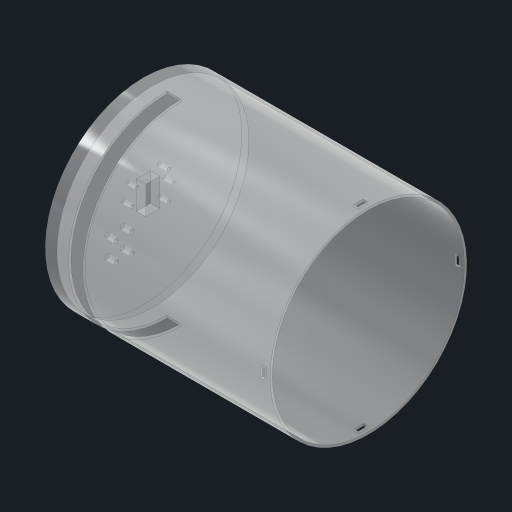
# Autodesk Inventor part: OUTK_001_ChipBucket
Saved by Autodesk Inventor 2024.2 (Build 282272000, 272)
## iProperties
Created: 2024-11-24
Part Number: OUTK_001_ChipBucket
Material: Polycarbonate, Clear
Document SubType Name: Modeling
Designer: Bryan
Density: 1.2 g/cm^3
Appearance: Polycarbonate - Clear
Mass: 1651.38 g
Surface Area: 5531.68 cm^2
Volume: 1376.15 cm^3
Author: Bryan
Autodesk Inventor part; units mm, degrees
ref_plane "YZ Plane" through (0, 0, 0) normal (1, 0, 0) x (0, 1, 0)
ref_plane "XZ Plane" through (0, 0, 0) normal (0, 1, 0) x (-1, 0, 0)
ref_plane "XY Plane" through (0, 0, 0) normal (0, 0, 1) x (1, 0, 0)
sketch "Sketch1" plane through (0, 0, 0) normal (1, 0, 0) x (0, 1, 0)
  circle A0 centre (0, 0) radius 133.35
  dimension "d0" = 266.7
  constraints: 1 centre point, 1 coincident
  measures "d0" diameter of A0
extrude "Extrusion1" add sketch "Sketch1" along normal mid plane 304.8
sketch "Sketch2" plane through (152.4, 0, 0) normal (1, 0, 0) x (0, 0, -1)
  circle A0 centre (0, 0) radius 130.175
  dimension "d3" = 260.35
  constraints: 1 centre point, 1 coincident
  measures "d3" diameter of A0
extrude "Extrusion2" cut sketch "Sketch2" against normal blind 292.1
sketch "Sketch3" plane through (0, 0, 0) normal (0, 0, 1) x (1, 0, 0)
  line L0 (-139.7, 130.175) -> (-139.7, -130.175) projected
  line L1 (152.4, 130.175) -> (152.4, -130.175) projected
  line L2 (152.4, 130.175) -> (-139.7, 130.175) projected
  line L3 (152.4, -130.175) -> (-139.7, -130.175) projected
  line L4 (-120.65, 130.175) -> (-120.65, -130.175)
  line L5 (-101.6, -130.175) -> (-101.6, 130.175)
  point P0 (0, 0)
  dimension "d6" = 19.05
  dimension "d7" = 19.05
  constraints: 4 end point, 4 point on line, 1 parallel, 1 vertical
  measures "d6" distance between parallel lines of L0 L4
  measures "d7" distance between parallel lines of L4 L5
extrude "Extrusion3" cut sketch "Sketch3" along normal blind 266.7 contours L2 L5 L3 L4
sketch "Sketch4" plane through (0, 0, 0) normal (0, 1, 0) x (-1, 0, 0)
  line L0 (120.65, 0) -> (101.6, 0) projected
  line L1 (120.65, 0) -> (120.65, 28.9256) projected
  line L2 (101.6, 0) -> (101.6, 28.9256) projected
  line L3 (101.6, 28.9256) -> (120.65, 28.9256) projected
  point P0 (0, 0)
extrude "Extrusion4" cut sketch "Sketch4" along normal through all both and the other way through all
sketch "Sketch5" plane through (0, 0, 0) normal (0, 1, 0) x (-1, 0, 0)
  line L0 (-139.065, 6.35) -> (-144.78, 6.35)
  line L1 (-144.78, 6.35) -> (-144.78, -6.35)
  line L2 (-144.78, -6.35) -> (-139.065, -6.35)
  line L3 (-139.065, -6.35) -> (-139.065, 6.35)
  line L4 (-152.4, 133.35) -> (-152.4, -133.35) projected
  point P0 (0, 0)
  point P1 (-139.065, 0)
  dimension "d12" = 5.715
  dimension "d13" = 12.7
  dimension "d14" = 7.62
  constraints: 8 end point, 2 parallel, 1 horizontal, 1 horizontal alignment, 1 midpoint, 1 perpendicular
  measures "d12" distance of L2.end L1.end
  measures "d13" distance of L1.end L0.end
  measures "d14" distance between parallel lines of L4 L1
extrude "Extrusion5" cut sketch "Sketch5" along normal through all both and the other way through all
sketch "Sketch6" plane through (0, 0, 0) normal (0, 0, 1) x (1, 0, 0)
  line L0 (139.065, 6.35) -> (144.78, 6.35)
  line L1 (144.78, 6.35) -> (144.78, -6.35)
  line L2 (144.78, -6.35) -> (139.065, -6.35)
  line L3 (139.065, -6.35) -> (139.065, 6.35)
  line L4 (152.4, -133.35) -> (152.4, 133.35) projected
  point P0 (0, 0)
  point P1 (139.065, 0)
  dimension "d17" = 5.715
  dimension "d18" = 12.7
  dimension "d19" = 7.62
  constraints: 8 end point, 2 parallel, 1 horizontal, 1 horizontal alignment, 1 midpoint, 1 perpendicular
  measures "d17" distance of L1.end L2.end
  measures "d18" distance of L0.end L1.end
  measures "d19" distance between parallel lines of L4 L1
extrude "Extrusion6" cut sketch "Sketch6" along normal through all both and the other way through all
sketch "Sketch8" plane through (-152.4, 0, 0) normal (-1, 0, 0) x (0, 0, 1)
  line L0 (-9.525, -19.05) -> (9.525, -19.05)
  line L1 (9.525, -19.05) -> (9.525, 19.05)
  line L2 (9.525, 19.05) -> (-9.525, 19.05)
  line L3 (-9.525, 19.05) -> (-9.525, -19.05)
  circle A0 centre (28.575, -27.1526) radius 3.2512
  circle A1 centre (28.575, -52.5526) radius 3.2512
  circle A2 centre (49.4284, -27.1526) radius 3.2512
  circle A3 centre (49.4284, -52.5526) radius 3.2512
  line L4 (-9.525, -14.4526) -> (9.525, -14.4526) construction
  line L5 (0, -14.4526) -> (0, -65.2526) construction
  line L6 (28.575, -27.1526) -> (28.575, -52.5526) construction
  line L7 (-6.35, -15.875) -> (-6.35, 15.875) construction
  line L8 (-6.35, 15.875) -> (6.35, 15.875) construction
  line L9 (6.35, 15.875) -> (6.35, -15.875) construction
  line L10 (6.35, -15.875) -> (-6.35, -15.875) construction
  line L11 (-6.35, -8.1026) -> (-2.3812, -4.1338) construction
  line L12 (-2.3812, -4.1338) -> (-2.3812, 8.5662) construction
  line L13 (6.35, 12.5349) -> (2.3813, 8.5662) construction
  line L14 (2.3813, 8.5662) -> (2.3813, -4.1338) construction
  line L15 (2.3813, -4.1338) -> (6.35, -8.1026) construction
  line L16 (0, -15.875) -> (0, 15.875) construction
  line L17 (-2.3812, 8.5662) -> (-6.35, 12.5349) construction
  line L18 (2.3813, 8.5662) -> (21.4312, 8.5662) construction
  line L19 (21.4312, 8.5662) -> (21.4312, -4.1339) construction
  line L20 (21.4312, -4.1339) -> (2.3813, -4.1338) construction
  line L21 (2.3813, -4.1338) -> (2.3813, 8.5662) construction
  line L22 (-2.3812, 8.5662) -> (-21.4312, 8.5661) construction
  line L23 (-21.4312, 8.5661) -> (-21.4312, -4.1338) construction
  line L24 (-21.4312, -4.1338) -> (-2.3812, -4.1338) construction
  line L25 (-2.3812, -4.1338) -> (-2.3812, 8.5662) construction
  line L26 (-15.0812, 14.9162) -> (-8.7312, 14.9162) construction
  line L27 (-8.7312, 14.9162) -> (-8.7312, -10.4839) construction
  line L28 (-8.7312, -10.4839) -> (-15.0812, -10.4839) construction
  line L29 (-15.0812, -10.4839) -> (-15.0812, 14.9162) construction
  line L30 (-21.4312, 2.2161) -> (-15.0812, 2.2161) construction
  circle A4 centre (-21.4312, -16.8338) radius 2.4892
  circle A5 centre (-27.7812, 2.2161) radius 2.4892
  circle A6 centre (-21.4312, 21.2662) radius 2.4892
  circle A7 centre (21.4312, -16.8338) radius 2.4892
  circle A8 centre (27.7812, 2.2161) radius 2.4892
  circle A9 centre (21.4312, 21.2662) radius 2.4892
  point P0 (0, 0)
  point P1 (28.575, -39.8526)
  point P2 (0, -39.8526)
  point P3 (-2.3813, 2.2162)
  point P4 (0, 0)
  point P5 (0, 19.05)
  point P6 (-9.525, 0)
  point P7 (-11.9062, 14.9162)
  point P8 (-11.9062, 8.5662)
  point P9 (-11.9062, -10.4839)
  point P10 (-18.2562, 2.2161)
  dimension "d22" = 19.05
  dimension "d23" = 38.1
  dimension "d24" = 6.5024
  dimension "d25" = 25.4
  dimension "d26" = 20.8534
  dimension "d28" = 19.05
  dimension "d31" = 4.5974
  dimension "d32" = 50.8
  dimension "d35" = 3.175
  dimension "d36" = 3.175
  dimension "d37" = 3.175
  dimension "d38" = 3.175
  dimension "d39" = 3.9688
  dimension "d40" = 12.7
  dimension "d41" = 45
  dimension "d42" = 45
  dimension "d44" = 19.05
  dimension "d45" = 6.35
  dimension "d46" = 25.4
  dimension "d47" = 7.7724
  dimension "d56" = 12.7
  dimension "d57" = 4.9784
  dimension "d58" = 6.35
  dimension "d59" = 19.05
  dimension "d60" = 6.35
  constraints: 62 end point, 15 midpoint, 10 centre point, 8 horizontal, 8 horizontal alignment, 8 parallel, 6 equal length, 6 point on line, 6 vertical, 5 vertical alignment, 4 equal radius, 4 perpendicular, 3 symmetric about line, 4 other
  measures "d22" distance of L2.end L1.end
  measures "d23" distance of L1.end L0.end
  measures "d24" diameter of A0
  measures "d25" distance of A3.centre A2.centre
  measures "d26" distance of A3.centre L6.end
  measures "d28" distance from line of L6.end L1
  measures "d31" distance between parallel lines of L0 L4
  measures "d32" distance of L5.start L5.end
  measures "d35" distance between parallel lines of L2 L8
  measures "d36" distance between parallel lines of L3 L7
  measures "d37" distance between parallel lines of L1 L9
  measures "d38" distance between parallel lines of L0 L10
  measures "d39" distance between parallel lines of L9 L14
  measures "d40" distance of L13.end L14.end
  measures "d41" angle of L11 L7
  measures "d42" angle of L7 L17
  measures "d44" distance of L12.end L22.end
  measures "d45" distance of L27.end L28.end
  measures "d46" distance of L28.end L26.start
  measures "d47" distance from line of L10 L15.end
  measures "d56" distance of A4.centre L23.end
  measures "d57" diameter of A4
  measures "d58" distance of A5.centre L30.start
  measures "d59" vertical distance of A4.centre A5.centre
  measures "d60" horizontal distance of A4.centre A5.centre
extrude "Extrusion7" cut sketch "Sketch8" against normal blind 25.4 contours L3 L2 L1 L0 | A0 | A1 | A2 | A3 | A4 | A5 | A6 | A8 | A9
body "Solid1"
